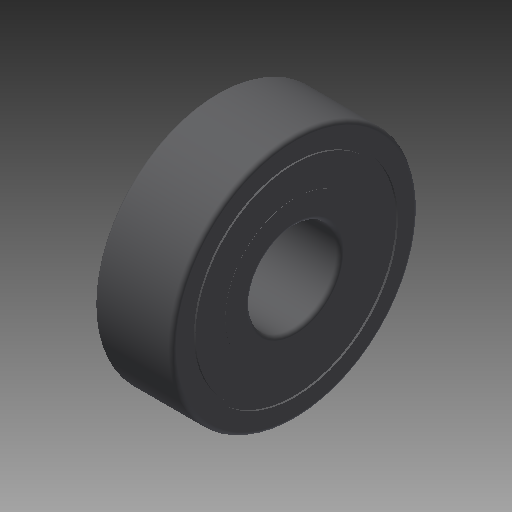
# Autodesk Inventor part: FF 10 Part2
Saved by Autodesk Inventor 2018 (Build 220112000, 112)
## iProperties
Category: PARTsolutions
Company: THK
Created: 2017-06-20
Part Number: FF 10 Part2
Catalog Web Link: www.cadenas.de
Description: Supported side type FF-P2-
Vendor: THK
Document SubType Name: Modeling
Designer: psAdmin
Manufacturer: THK
Mass: 2.29361 g
Surface Area: 13.2688 cm^2
Volume: 2.29361 cm^3
Density: 1 g/cm^3
Material: Generic
Appearance: PSOLRGB-192-192-192
PSOL_IDENT_0: {$CADENAS_DATA\23d-libs\thk\fed_screw\ball_screw\ball_screw_peripheral\suport_unit\supported_ff_2.pr
PSOL_IDENT_1: j},183 {VTYP=3D},{NB=FF 10 Part2},{LINA=FF 10 Part2},{NN=Supported side type FF-P2},{DATE=02.06.2017
PSOL_IDENT_2: 06:41:21},{GEOMDATE=02.02.2010 00:00:00},{VERSION=},{LINEID=20},{LINESUBID=-1},{WBVAR=}  {NB=FF 10
PSOL_IDENT_3: Part2},{LINA=FF 10 Part2},{KT=DUMMY},{IDNR=},{MN=FF 10},{SDX=22.000},{LX=7.000},{SD=8.000},{D1=18.40
PSOL_IDENT_4: 0},{D2=17.800},{D3=12.500}
NN: Supported side type FF-P2
NB: FF 10 Part2
NBSYN: $MN. Part2
LINA: FF 10 Part2
MN: FF 10
SDX: 22.000
LX: 7.000
SD: 8.000
D1: 18.400
D2: 17.800
D3: 12.500
SUPPLIER: THK
ARTICLENO: FF 10 Part2
BOMINFO: FF 10 Part2
CREATOR: CADENAS GmbH
Title: FF 10 Part2
Author: Cadenas PARTsolutions
Autodesk Inventor part; units mm, degrees
sketch "Sketch_1" plane through (0, 0, 0) normal (0, 0, 1) x (1, 0, 0)
  line L0 (50, 0) -> (-50, 0)
  arc A0 (-3.5, 4.35) -> (-3.15, 4) centre (-3.15, 4.35) ccw
  line L1 (-3.15, 4) -> (3.15, 4)
  arc A1 (3.15, 4) -> (3.5, 4.35) centre (3.15, 4.35) ccw
  line L2 (3.5, 4.35) -> (3.5, 10.65)
  arc A2 (3.5, 10.65) -> (3.15, 11) centre (3.15, 10.65) ccw
  line L3 (3.15, 11) -> (-3.15, 11)
  arc A3 (-3.15, 11) -> (-3.5, 10.65) centre (-3.15, 10.65) ccw
  line L4 (-3.5, 10.65) -> (-3.5, 4.35)
  constraints: 10 end point, 8 point on circle, 4 centre point
revolve "Revolution1" add sketch "Sketch_1" angle 360 about axis through (50, 0, 0) along (1, 0, 0)
sketch "Sketch_2" plane through (0, 0, 0) normal (0, 0, 1) x (1, 0, 0)
  line L0 (50, 0) -> (-50, 0)
  line L1 (-5.34, 9.2) -> (-5.34, 4)
  line L2 (-5.34, 4) -> (-3.5, 4)
  line L3 (-3.5, 4) -> (-3.5, 6.25)
  line L4 (-3.5, 6.25) -> (-3.48, 6.25)
  line L5 (-3.48, 6.25) -> (-3.48, 8.9)
  line L6 (-3.48, 8.9) -> (-3.34, 8.9)
  line L7 (-3.34, 8.9) -> (-3.34, 9.2)
  line L8 (-3.34, 9.2) -> (-5.34, 9.2)
  constraints: 18 end point
revolve "Revolution2" cut sketch "Sketch_2" angle 360 about axis through (50, 0, 0) along (1, 0, 0)
sketch "Sketch_3" plane through (0, 0, 0) normal (0, 0, 1) x (1, 0, 0)
  line L0 (50, 0) -> (-50, 0)
  line L1 (3.34, 8.9) -> (3.48, 8.9)
  line L2 (3.48, 8.9) -> (3.48, 6.25)
  line L3 (3.48, 6.25) -> (3.5, 6.25)
  line L4 (3.5, 6.25) -> (3.5, 4)
  line L5 (3.5, 4) -> (5.34, 4)
  line L6 (5.34, 4) -> (5.34, 9.2)
  line L7 (5.34, 9.2) -> (3.34, 9.2)
  line L8 (3.34, 9.2) -> (3.34, 8.9)
  constraints: 18 end point
revolve "Revolution3" cut sketch "Sketch_3" angle 360 about axis through (50, 0, 0) along (1, 0, 0)
ref_plane "ff_2_XY" through (0, 0, 0) normal (1, 0, 0) x (0, 0, -1)
ref_plane "ff_2_YZ" through (0, 0, 0) normal (0, 0, -1) x (0, 1, 0)
ref_plane "ff_2_ZX" through (0, 0, 0) normal (0, 1, 0) x (1, 0, 0)
body "Solid1"
